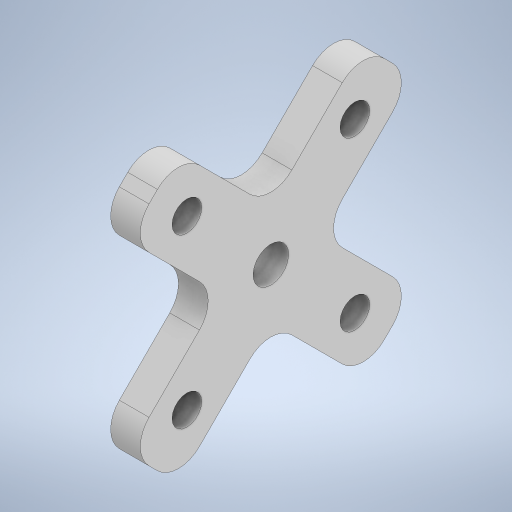
# Autodesk Inventor part: Gearbox
Saved by Autodesk Inventor 2023 (Build 270158000, 158)
## iProperties
Created: 2024-01-10
Part Number: Gearbox
Material: Generic
Document SubType Name: Modeling
Designer: thesl
Density: 1 g/cm^3
Appearance: Default
Author: thesl
Autodesk Inventor part; units mm, degrees
ref_plane "YZ Plane" through (0, 0, 0) normal (1, 0, 0) x (0, 1, 0)
ref_plane "XZ Plane" through (0, 0, 0) normal (0, 1, 0) x (-1, 0, 0)
ref_plane "XY Plane" through (0, 0, 0) normal (0, 0, 1) x (1, 0, 0)
sketch "Sketch1" plane through (0, 0, 0) normal (1, 0, 0) x (0, 1, 0)
  circle A0 centre (17.9578, -17.9578) radius 3.81
  circle A1 centre (35.9156, 0) radius 3.175
  circle A2 centre (0, -35.9156) radius 3.175
  circle A3 centre (35.9156, -35.9156) radius 3.175
  circle A4 centre (0, 0) radius 3.175
  line L0 (17.9578, -17.9578) -> (23.346, -23.346)
  line L1 (23.346, -23.346) -> (12.5696, -23.346)
  line L2 (17.9578, -28.7341) -> (37.7144, -48.4907)
  line L3 (37.7144, -48.4907) -> (48.4907, -37.7144)
  line L4 (48.4907, -37.7144) -> (28.7341, -17.9578)
  line L5 (17.9578, -28.7341) -> (-1.7988, -48.4907)
  line L6 (-1.7988, -48.4907) -> (-12.5751, -37.7144)
  line L7 (-12.5751, -37.7144) -> (7.1815, -17.9578)
  line L8 (7.1815, -17.9578) -> (-12.5751, 1.7988)
  line L9 (-12.5751, 1.7988) -> (-1.7988, 12.5751)
  line L10 (-1.7988, 12.5751) -> (17.9578, -7.1815)
  line L11 (17.9578, -7.1815) -> (37.7144, 12.5751)
  line L12 (37.7144, 12.5751) -> (48.4907, 1.7988)
  line L13 (48.4907, 1.7988) -> (28.7341, -17.9578)
  line L14 (35.9156, 0) -> (33.6705, -2.2451)
  line L15 (0, 0) -> (2.2451, -2.2451)
  line L16 (15.2637, -15.2637) -> (17.9578, -17.9578)
  line L17 (22.6724, -13.2432) -> (20.6519, -15.2637)
  line L18 (15.2637, -20.6519) -> (12.5696, -23.346)
  line L19 (2.2451, -33.6705) -> (0, -35.9156)
  line L20 (35.9156, 0) -> (35.9156, -3.175)
  line L21 (35.9156, -32.7406) -> (35.9156, -35.9156)
  line L22 (35.9156, -35.9156) -> (32.7406, -35.9156)
  line L23 (3.175, -35.9156) -> (0, -35.9156)
  line L24 (0, -35.9156) -> (0, -32.7406)
  line L25 (0, -3.175) -> (0, 0)
  line L26 (0, 0) -> (3.175, 0)
  line L27 (32.7406, 0) -> (35.9156, 0)
  point P0 (20.6519, -20.6519)
  dimension "d0" = 35.9156
  dimension "d1" = 35.9156
  dimension "d2" = 7.62
  dimension "d3" = 6.35
  dimension "d4" = 6.35
  dimension "d5" = 6.35
  dimension "d6" = 6.35
  dimension "d7" = 7.62
  dimension "d8" = 35.56
  dimension "d9" = 15.24
  dimension "d10" = 35.56
  dimension "d11" = 15.24
  dimension "d12" = 35.56
  constraints: 56 end point, 16 perpendicular, 14 point on circle, 10 parallel, 5 centre point, 4 coincident, 4 point on line, 3 horizontal
  measures "d0" distance of L21.end L19.end
  measures "d1" distance of L14.start L21.end
  measures "d2" diameter of A0
  measures "d3" diameter of A1
  measures "d4" diameter of A2
  measures "d5" diameter of A3
  measures "d6" diameter of A4
  measures "d7" distance of L0.start L0.end
  measures "d8" distance of L1.end L2.end
  measures "d9" distance of L2.end L3.end
  measures "d10" distance of L0.end L5.end
  measures "d11" distance of L5.end L6.end
  measures "d12" distance of L1.end L8.end
extrude "Extrusion1" add sketch "Sketch1" along normal blind 6.35 contours L0 L1 L18 A0 | L5 L6 L7 L8 L9 L10 L11 L12 L13 L4 L3 L2
fillet "Fillet1" radius 6.35 12 edges at (3.175, 28.7341, -17.9578) (3.175, 48.4907, -37.7144) (3.175, 37.7144, -48.4907) (3.175, -1.7988, -48.4907) (3.175, -1.7988, 12.5751) (3.175, 37.7144, 12.5751) (3.175, 48.4907, 1.7988) (3.175, 17.9578, -28.7341) (3.175, -12.5751, -37.7144) (3.175, -12.5751, 1.7988) (3.175, 7.1815, -17.9578) (3.175, 17.9578, -7.1815)
body "Solid1"
